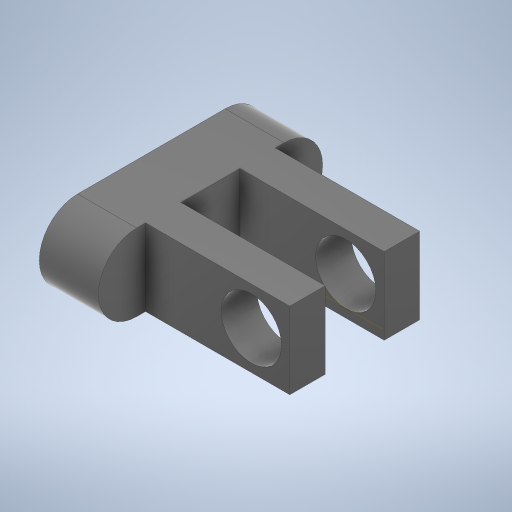
# Autodesk Inventor part: ObenMotor
Saved by Autodesk Inventor 2023 (Build 270158000, 158)
## iProperties
Created: 2024-01-25
Part Number: ObenMotor
Material: Generisch
Document SubType Name: Modeling
Designer: phili
Density: 1 g/cm^3
Appearance: Vorgabe
Author: phili
Autodesk Inventor part; units mm, degrees
ref_plane "YZ Plane" through (0, 0, 0) normal (1, 0, 0) x (0, 1, 0)
sketch "Skizze1" plane through (0, 0, 0) normal (1, 0, 0) x (0, 1, 0)
  circle A0 centre (0, 12.5) radius 6.5
  circle A1 centre (0, -12.5) radius 6.5
  line L0 (6.5, 12.5) -> (6.5, -12.5)
  line L1 (-6.5, -12.5) -> (-6.5, 12.5)
  point P0 (0, 0)
  dimension "d0" = 13
  dimension "d1" = 13
  dimension "d2" = 12.5
  dimension "d3" = 12.5
  constraints: 4 end point, 4 point on circle, 2 centre point, 2 tangent, 1 parallel
  measures "d0" diameter of A0
  measures "d1" diameter of A1
  measures "d2" distance of point (0, 0) A0.centre
  measures "d3" distance of A1.centre point (0, 0)
extrude "Extrusion1" add sketch "Skizze1" along normal blind 10
sketch "Skizze2" plane through (0, 0, 0) normal (-1, 0, 0) x (0, 0, 1)
  arc A0 (-12.5, 6.5) -> (-12.5, -6.5) centre (-12.5, 0) ccw projected
  circle A1 centre (-12.5, 0) radius 5.05
  arc A2 (12.5, -6.5) -> (12.5, 6.5) centre (12.5, 0) ccw projected
  circle A3 centre (12.5, 0) radius 5.05
  point P0 (0, 0)
  dimension "d8" = 10.1
  dimension "d9" = 10.1
  constraints: 2 centre point, 2 coincident
  measures "d8" diameter of A1
  measures "d9" diameter of A3
extrude "Extrusion2" cut sketch "Skizze2" against normal blind 6
ref_plane "Arbeitsebene1" through (0, 0, 5) normal (0, 0, 1) x (1, 0, 0)
sketch "Skizze4" plane through (0, 0, 5) normal (0, 0, 1) x (1, 0, 0)
  line L0 (10, -6.5) -> (10, 6.5) projected
  line L1 (27.9456, 6.5) -> (10, 6.5)
  line L2 (27.9456, -6.5) -> (10, -6.5)
  line L3 (0, -6.5) -> (0, 6.5) projected
  line L4 (27.9456, 6.5) -> (34.4456, 6.5)
  line L5 (34.4456, 6.5) -> (34.4456, -6.5)
  line L6 (34.4456, -6.5) -> (27.9456, -6.5)
  point P0 (0, 0)
  point P1 (0, 0)
  constraints: 10 end point, 2 point on line, 1 midpoint, 1 perpendicular
extrude "Extrusion3" add sketch "Skizze4" along normal blind 6
ref_plane "Arbeitsebene2" through (0, 0, -5) normal (0, 0, 1) x (1, 0, 0)
sketch "Skizze5" plane through (0, 0, -5) normal (0, 0, 1) x (1, 0, 0)
  line L0 (34.4456, 6.5) -> (10, 6.5) projected
  line L1 (10, 6.5) -> (10, -6.5) projected
  line L2 (27.9456, 6.5) -> (10, 6.5)
  line L3 (10, -6.5) -> (34.4456, -6.5) projected
  line L4 (27.9456, -6.5) -> (10, -6.5)
  line L5 (34.4456, -6.5) -> (34.4456, 6.5) projected
  line L6 (27.9456, 6.5) -> (34.4456, 6.5)
  line L7 (34.4456, 6.5) -> (34.4456, -6.5)
  line L8 (34.4456, -6.5) -> (27.9456, -6.5)
  point P0 (0, 0)
  point P1 (27.9456, 0)
  dimension "d26" = 24.4456
  dimension "d27" = 13
  constraints: 10 end point, 1 collinear, 1 perpendicular
  measures "d26" distance of L0.start L0.end
  measures "d27" distance of L3.end L0.start
extrude "Extrusion4" add sketch "Skizze5" against normal blind 6
sketch "Skizze6" plane through (0, 0, -11) normal (0, 0, -1) x (-1, 0, 0)
  arc A0 (-27.9456, 6.5) -> (-27.9456, -6.5) centre (-27.9456, 0) ccw projected
  circle A1 centre (-27.9456, 0) radius 5.1
  point P0 (0, 0)
  dimension "d20" = 10.2
  constraints: 1 centre point, 1 coincident
  measures "d20" diameter of A1
extrude "Extrusion5" cut sketch "Skizze6" against normal through all
ref_plane "Arbeitsebene3" through (0, 0, 0) normal (0, 1, 0) x (-1, 0, 0)
ref_plane "Arbeitsebene4" through (0, 0, 0) normal (0, 0, 1) x (1, 0, 0)
